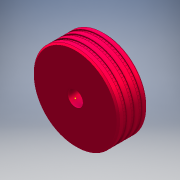
# Autodesk Inventor part: Part4
Saved by Autodesk Inventor 2016 (Build 200138000, 138)
## iProperties
Created: 2016-09-09
Part Number: Part4
Material: Generic
Document SubType Name: Modeling
Designer: Muhammad
Density: 1 g/cm^3
Appearance: Default
Author: Muhammad
Autodesk Inventor part; units mm, degrees
ref_plane "YZ Plane" through (0, 0, 0) normal (1, 0, 0) x (0, 1, 0)
ref_plane "XZ Plane" through (0, 0, 0) normal (0, 1, 0) x (-1, 0, 0)
sketch "Sketch1" plane through (0, 0, 0) normal (0, 1, 0) x (-1, 0, 0)
  circle A0 centre (0, 0) radius 14
  circle A1 centre (0, 0) radius 2.5
  dimension "d0" = 28
  dimension "d1" = 5
  constraints: 2 centre point, 2 coincident
  measures "d0" diameter of A0
  measures "d1" diameter of A1
extrude "Extrusion1" add sketch "Sketch1" along normal blind 9.5
sketch "Sketch2" plane through (0, 0, 0) normal (0, 0, 1) x (1, 0, 0)
  point P0 (0, 0)
ref_plane "Work Plane2" through (0, 0, 13.7) normal (0, 0, 1) x (1, 0, 0)
sketch "Sketch4" plane through (0, 0, 13.7) normal (0, 0, 1) x (1, 0, 0)
  line L0 (0, 0) -> (0, 2.25) construction
  line L1 (0, 2.25) -> (0, 7.25) construction
  line L2 (-2.5, 0) -> (-2.5, 9.5) construction
  line L3 (-2.5, 4.75) -> (2.2172, 4.75) construction
  line L4 (-2.5, 4.75) -> (-2.5, 4.25)
  line L5 (-2.5, 4.25) -> (2.2172, 4.25)
  line L6 (2.5, 0) -> (2.5, 9.5) projected
  line L7 (2.2172, 4.25) -> (2.2172, 5.25)
  line L8 (2.2172, 5.25) -> (-2.5, 5.25)
  line L9 (-2.5, 4.75) -> (-2.5, 5.25)
  line L10 (2.2172, 2.25) -> (2.2172, 1.75)
  line L11 (2.2172, 1.75) -> (-2.5, 1.75)
  line L12 (-2.5, 1.75) -> (-2.5, 2.75)
  line L13 (-2.5, 2.75) -> (2.2172, 2.75)
  line L14 (2.2172, 2.75) -> (2.2172, 2.25)
  line L15 (2.2172, 7.25) -> (2.2172, 7.75)
  line L16 (2.2172, 7.75) -> (-2.5, 7.75)
  line L17 (-2.5, 7.75) -> (-2.5, 6.75)
  line L18 (-2.5, 6.75) -> (2.2172, 6.75)
  line L19 (2.2172, 6.75) -> (2.2172, 7.25)
  dimension "d26" = 1
  dimension "d28" = 1
  constraints: 36 end point, 7 point on line, 6 perpendicular, 5 symmetric about line, 2 vertical, 1 collinear, 1 horizontal, 1 midpoint
  measures "d26" distance of L5.end L7.end
  measures "d28" distance of L11.end L12.end
extrude "Extrusion3" cut sketch "Sketch4" along normal through all
pattern_circular "Circular Pattern2" count 90 over 360 about axis through (0, 0, 0) along (0, 1, 0) of "Extrusion3"
chamfer "Chamfer2" distance 0.5 angle 45 2 edges at (14, 0, 0) (14, 9.5, 0)
body "Solid1"
